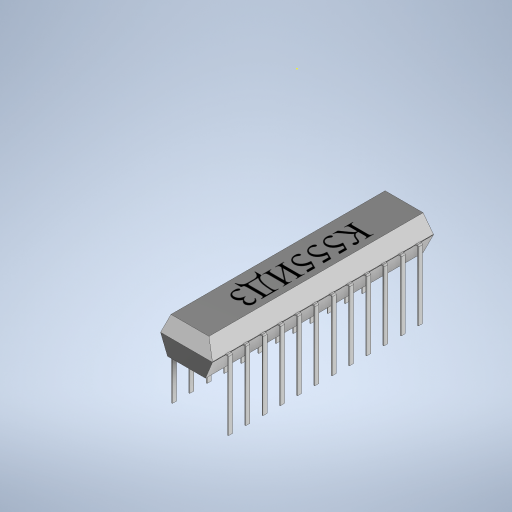
# Autodesk Inventor part: К555ИД3
Saved by Autodesk Inventor 2024 (Build 280153000, 153)
## iProperties
Created: 2023-12-04
Part Number: К555ИД3
Material: Типовые
Document SubType Name: Modeling
Designer: SaNe4Ka
Density: 1 g/cm^3
Appearance: По умолчанию
Author: SaNe4Ka
Autodesk Inventor part; units mm, degrees
ref_plane "YZ Plane" through (0, 0, 0) normal (1, 0, 0) x (0, 1, 0)
ref_plane "XZ Plane" through (0, 0, 0) normal (0, 1, 0) x (-1, 0, 0)
ref_plane "XY Plane" through (0, 0, 0) normal (0, 0, 1) x (1, 0, 0)
sketch "Эскиз1" plane through (0, 0, 0) normal (0, 1, 0) x (-1, 0, 0)
  line L0 (-20.6985, 40.4468) -> (-28.1985, 40.4468)
  line L1 (-28.1985, 40.4468) -> (-28.1985, 8.4468)
  line L2 (-28.1985, 8.4468) -> (-20.6985, 8.4468)
  line L3 (-20.6985, 8.4468) -> (-20.6985, 40.4468)
  point P0 (0, 0)
  dimension "d0" = 7.5
  dimension "d1" = 32
  constraints: 8 end point, 2 parallel, 1 horizontal, 1 perpendicular
  measures "d0" distance of L2.end L1.end
  measures "d1" distance of L1.end L0.end
extrude "Выдавливание2" add sketch "Эскиз1" along normal blind 5
ref_plane "РабПлоскость2" through (20.6985, 0, 8.4468) normal (-1, 0, 0) x (0, 0, 1)
sketch "Эскиз3" plane through (20.6985, 0, 8.4468) normal (-1, 0, 0) x (0, 0, 1)
  line L0 (32, 0) -> (32, 5) projected
  line L1 (30.05, 2.565) -> (30.05, 2.435)
  line L2 (30.05, 2.435) -> (29.45, 2.435)
  line L3 (29.45, 2.435) -> (29.45, 2.565)
  line L4 (29.45, 2.565) -> (30.05, 2.565)
  point P0 (-8.4468, 0)
  dimension "d23" = 0.6
  constraints: 8 end point, 2 perpendicular, 1 horizontal
  measures "d23" distance of L1.end L2.end
ref_plane "РабПлоскость3" through (20.6985, 0, 38.1968) normal (0, 0, 1) x (1, 0, 0)
sketch "Эскиз4" plane through (20.6985, 0, 38.1968) normal (0, 0, 1) x (1, 0, 0)
  line L0 (0, 0) -> (0, 5) projected
  line L1 (0, 2.5) -> (-0.2, 2.5)
  line L2 (-0.3, 2.4) -> (-0.3, -7.5)
  arc A0 (-0.2, 2.5) -> (-0.3, 2.4) centre (-0.2, 2.4) ccw
  point P0 (-20.6985, 0)
  point P1 (-0.3, 2.5)
  dimension "d24" = 0.3
  dimension "d25" = 10
  dimension "d26" = 0.1
  constraints: 4 end point, 2 point on circle, 2 point on line, 2 tangent, 1 centre point, 1 horizontal, 1 midpoint, 1 perpendicular
  measures "d24" distance of L1.start point (-0.3, 2.5)
  measures "d25" distance of point (-0.3, 2.5) L2.end
  measures "d26" radius of A0
sweep "Сдвиг2" add profiles "Эскиз3" path "Эскиз4" path curves L1 A0 L2
ref_plane "РабПлоскость4" through (28.1985, 0, 40.4468) normal (1, 0, 0) x (0, 0, -1)
sketch "Эскиз5" plane through (28.1985, 0, 40.4468) normal (1, 0, 0) x (0, 0, -1)
  line L0 (0, 0) -> (0, 5) projected
  line L1 (1.95, 2.435) -> (2.55, 2.435) projected
  line L2 (2.55, 2.435) -> (2.55, 2.565)
  line L3 (1.95, 2.435) -> (2.55, 2.435)
  line L4 (1.95, 2.565) -> (1.95, 2.435) projected
  line L5 (1.95, 2.435) -> (1.95, 2.565)
  line L6 (2.55, 2.565) -> (1.95, 2.565) projected
  line L7 (1.95, 2.565) -> (2.55, 2.565)
  point P0 (40.4468, 0)
  constraints: 8 end point, 2 vertical, 1 collinear, 1 perpendicular
sketch "Эскиз6" plane through (20.6985, 0, 38.1968) normal (0, 0, 1) x (1, 0, 0)
  line L0 (7.5, 0) -> (7.5, 5) projected
  line L1 (7.5, 2.5) -> (7.7, 2.5)
  line L2 (7.8, 2.4) -> (7.8, -7.5)
  arc A0 (7.8, 2.4) -> (7.7, 2.5) centre (7.7, 2.4) ccw
  point P0 (-20.6985, 0)
  point P1 (7.8, 2.5)
  dimension "d35" = 0.3
  dimension "d36" = 10
  dimension "d37" = 0.1
  constraints: 4 end point, 2 point on circle, 2 point on line, 2 tangent, 1 centre point, 1 horizontal, 1 midpoint, 1 perpendicular
  measures "d35" distance of L1.start point (7.8, 2.5)
  measures "d36" distance of point (7.8, 2.5) L2.end
  measures "d37" radius of A0
sweep "Сдвиг3" add profiles "Эскиз5" path "Эскиз6" path curves L1 A0 L2
pattern_linear "Прямоуг.массив1" count 12 spacing -2.5 along (0, 0, 1) of "Сдвиг2", "Сдвиг3"
chamfer "Фаска1" distance 0.5 distance2 2.5 1 edges at (24.4485, 5, 40.4468) measured on face at (24.4485, 5, 39.9468)
chamfer "Фаска2" distance 0.5 distance2 2.5 3 edges at (24.4485, 5, 8.4468) (28.1985, 5, 24.1968) (20.6985, 5, 24.1968) measured on face at (24.4485, 5, 8.9468) measured on face at (27.6985, 5, 24.1968) measured on face at (21.1985, 5, 24.1968)
chamfer "Фаска3" distance 2.5 distance2 0.5 1 edges at (24.4485, 0, 8.4468) measured on face at (24.4485, 0.5, 8.4468)
chamfer "Фаска4" distance 2.5 distance2 0.5 1 edges at (28.1985, 0, 24.6967) measured on face at (28.1985, 0.5, 24.6967)
chamfer "Фаска5" distance 2.5 distance2 0.5 1 edges at (20.6985, 0, 24.6967) measured on face at (20.6985, 0.5, 24.6967)
chamfer "Фаска6" distance 2.5 distance2 0.5 1 edges at (27.6985, 5, 24.4468) measured on face at (27.7966, 4.5097, 24.4468)
chamfer "Фаска7" distance 2.5 distance2 0.5 1 edges at (27.6985, 0, 24.6967) measured on face at (27.7966, 0.4903, 24.6967)
chamfer "Фаска8" distance 2.5 distance2 0.5 1 edges at (21.1985, 0, 24.6967) measured on face at (21.1005, 0.4903, 24.6967)
chamfer "Фаска9" distance 2.5 distance2 0.5 1 edges at (21.1985, 5, 24.4468) measured on face at (21.1005, 4.5097, 24.4468)
sketch "Эскиз7" plane through (0, 5, 0) normal (0, 1, 0) x (1, 0, 0)
  line L0 (26.3913, -15.1122) -> (26.3913, -33.8732) construction
  line L1 (26.3913, -33.8732) -> (22.4019, -33.8732) construction
  line L2 (22.4019, -33.8732) -> (22.4019, -15.1122) construction
  line L3 (22.4019, -15.1122) -> (26.3913, -15.1122) construction
  point P0 (0, 0)
  constraints: 2 other
